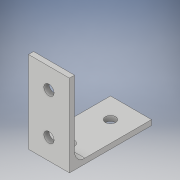
# Autodesk Inventor part: 2in 4-hole Bracket 0.25in Hole
Saved by Autodesk Inventor 2018 (Build 220112000, 112)
## iProperties
Created: 2020-02-16
Part Number: 2in 4-hole Bracket 0.25in Hole
Material: Generic
Document SubType Name: Modeling
Designer: T3500STATIC
Density: 1 g/cm^3
Appearance: Default
Author: T3500STATIC
Autodesk Inventor part; units mm, degrees
ref_plane "YZ Plane" through (0, 0, 0) normal (1, 0, 0) x (0, 1, 0)
ref_plane "XZ Plane" through (0, 0, 0) normal (0, 1, 0) x (-1, 0, 0)
ref_plane "XY Plane" through (0, 0, 0) normal (0, 0, 1) x (1, 0, 0)
sketch "Sketch1" plane through (0, 0, 0) normal (1, 0, 0) x (0, 1, 0)
  line L0 (0, 0) -> (50.8, 0)
  line L1 (50.8, 0) -> (50.8, -3.175)
  line L2 (50.8, -3.175) -> (0, -3.175)
  line L3 (0, -3.175) -> (0, 0)
  line L4 (0, 0) -> (3.175, 0)
  line L5 (3.175, 0) -> (3.175, -50.8)
  line L6 (3.175, -50.8) -> (0, -50.8)
  line L7 (0, -50.8) -> (0, 0)
  dimension "d0" = 50.8
  dimension "d1" = 3.175
  dimension "d2" = 3.175
  dimension "d3" = 50.8
  constraints: 16 end point, 4 parallel, 2 horizontal, 2 perpendicular
  measures "d0" distance of L1.end L2.end
  measures "d1" distance of L0.end L1.end
  measures "d2" distance of L5.end L6.end
  measures "d3" distance of L4.end L5.end
extrude "Extrusion1" add sketch "Sketch1" along normal blind 25.4
fillet "Fillet1" radius 6.35 1 edges at (12.7, 3.175, -3.175)
hole "Hole1" at (12.7, 0, -12.7) direction (0, 1, 0) diameter 6.35 end through all
hole "Hole2" at (12.7, 0, -38.1) direction (0, 1, 0) diameter 6.35 end through all
hole "Hole3" at (12.7, 12.7, 0) direction (0, 0, -1) diameter 6.35 end through all
hole "Hole4" at (12.7, 38.1, 0) direction (0, 0, -1) diameter 6.35 end through all
body "Solid1"
